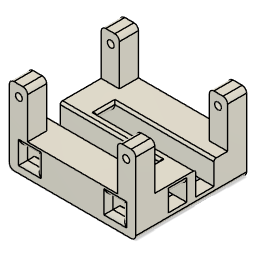
servoFrameMaking (Autodesk Fusion 360 design; units mm, degrees)
Autodesk Fusion 360 part; units mm, degrees
sketch "Sketch1" plane through (0, 0, 0) normal (1, 0, 0) x (0, 0, -1)
  line L0 (0, 0) -> (0, 7)
  line L1 (0, 7) -> (-1, 7)
  line L2 (-1, 7) -> (-1, 1.8)
  line L3 (-1, 1.8) -> (-5, 1.8)
  line L4 (-5, 1.8) -> (-5, 7)
  line L5 (-5, 7) -> (-12.2, 7)
  line L6 (-12.2, 7) -> (-12.2, 0)
  line L7 (-12.2, 0) -> (0, 0)
  dimension "d1" = 7
  dimension "d2" = 1
  dimension "d3" = 5.2
  dimension "d4" = 4
  dimension "d5" = 5.2
  dimension "d6" = 7.2
  dimension "d7" = 7
  constraint coincident L0.start L7.end
  constraint vertical L0
  constraint perpendicular L0 L1
  constraint perpendicular L1 L2
  constraint perpendicular L2 L3
  constraint perpendicular L3 L4
  constraint perpendicular L4 L5
  constraint perpendicular L5 L6
  measures "d1" distance of L0.start L0.end
  measures "d2" distance of L0.end L1.end
  measures "d3" distance of L1.end L2.end
  measures "d4" distance of L2.end L3.end
  measures "d5" distance of L3.end L4.end
  measures "d6" distance of L4.end L5.end
  measures "d7" distance of L5.end L6.end
extrude "Extrude1" add sketch "Sketch1" along normal blind 13.9 and the other way blind 13.9 makes body 1
sketch "Sketch2" plane through (0, 7, 0) normal (0, 1, 0) x (-1, 0, 0)
  line L0 (13.9, 12.2) -> (-13.9, 12.2)
  line L1 (-13.9, 12.2) -> (-13.9, 5)
  line L2 (-13.9, 5) -> (13.9, 5)
  line L3 (13.9, 5) -> (13.9, 12.2)
  line L4 (13.9, 12.2) -> (9.9, 12.2)
  line L5 (9.9, 12.2) -> (9.9, 8)
  line L6 (9.9, 8) -> (13.9, 8)
  line L7 (13.9, 8) -> (13.9, 12.2)
  dimension "d12" = 4
  dimension "d13" = 4.2
  constraint horizontal L4
  constraint vertical L5
  constraint horizontal L6
  constraint vertical L7
  constraint coincident L0.start L3.end
  measures "d12" distance of L0.start L4.end
  measures "d13" distance of L0.start L6.end
extrude "Extrude2" add sketch "Sketch2" along normal blind 10 separate body contours L0 L3 L4 L5 L6 L7 makes body 2
sketch "Sketch3" plane through (0, 0, 12.2) normal (0, 0, 1) x (1, 0, 0)
  line L0 (-13.9, 7) -> (-9.9, 7)
  line L1 (-9.9, 7) -> (-9.9, 17)
  line L2 (-9.9, 17) -> (-13.9, 17)
  line L3 (-13.9, 17) -> (-13.9, 7)
  line L4 (-13.9, 7) -> (-11.8, 7) construction
  line L5 (-11.8, 7) -> (-11.8, 14.6) construction
  line L6 (-11.8, 14.6) -> (-13.9, 14.6) construction
  line L7 (-13.9, 14.6) -> (-13.9, 7) construction
  circle A0 centre (-11.8, 14.6) radius 0.75
  dimension "d16" = 2.1
  dimension "d17" = 7.6
  dimension "d18" = 1.5
  constraint horizontal L4
  constraint vertical L5
  constraint horizontal L6
  constraint vertical L7
  constraint coincident L0.start L3.end
  constraint coincident L5.end L6.start
  measures "d16" distance of L0.start L4.end
  measures "d17" distance of L0.start L6.end
  measures "d18" diameter of A0
extrude "Extrude3" cut sketch "Sketch3" against normal blind 10 contours A0 bodies 2
fillet "Fillet1" radius 1 1 edges at (-13.9, 17, 10.1) on bodies 2
fillet "Fillet2" radius 1 1 edges at (-9.9, 17, 10.1) on bodies 2
mirror "Mirror1" about plane through (0, 0, 0) normal (1, 0, 0) of bodies 2 makes body 3
sketch "Sketch4" plane through (0, 0, 5) normal (0, 0, -1) x (-1, 0, 0)
  line L0 (13.9, 7) -> (-13.9, 7)
  line L1 (-13.9, 7) -> (-13.9, 1.8)
  line L2 (-13.9, 1.8) -> (13.9, 1.8)
  line L3 (13.9, 1.8) -> (13.9, 7)
  line L4 (-13.9, 7) -> (-7.9, 7)
  line L5 (-7.9, 7) -> (-7.9, 6.5)
  line L6 (-9.4, 5) -> (-12.4, 5)
  line L7 (-13.9, 6.5) -> (-13.9, 7)
  arc A0 (-9.4, 5) -> (-7.9, 6.5) centre (-9.4, 6.5) ccw
  arc A1 (-13.9, 6.5) -> (-12.4, 5) centre (-12.4, 6.5) ccw
  point P0 (-13.9, 5)
  dimension "d27" = 6
  dimension "d28" = 2
  dimension "d29" = 1.5
  dimension "d30" = 1.5
  constraint horizontal L4
  constraint vertical L5
  constraint horizontal L6
  constraint vertical L7
  constraint coincident L0.end L1.start
  constraint tangent L5 A0
  constraint tangent L6 A0
  constraint coincident P0 L6
  constraint coincident P0 L7
  constraint tangent L6 A1
  constraint tangent L7 A1
  measures "d27" distance of L0.end L4.end
  measures "d28" distance of L0.end P0
  measures "d29" radius of A0
  measures "d30" radius of A1
extrude "Extrude4" add sketch "Sketch4" along normal blind 4 contours L0 L1 L4 L5 L6 L7 A0 A1 bodies 1
sketch "Sketch5" plane through (13.9, 0, 0) normal (1, 0, 0) x (0, 0, -1)
  line L0 (0, 7) -> (-12.2, 7)
  line L1 (-12.2, 7) -> (-12.2, 0)
  line L2 (-12.2, 0) -> (0, 0)
  line L3 (0, 0) -> (0, 7)
  line L4 (-5, 6.5) -> (-1, 6.5)
  line L5 (-1, 6.5) -> (-1, 1.8)
  line L6 (-1, 1.8) -> (-5, 1.8)
  line L7 (-5, 1.8) -> (-5, 6.5)
  line L8 (-1, 1.8) -> (0, 1.8)
  line L9 (-5, 1.8) -> (-6, 1.8)
  line L10 (-12.2, 0) -> (-12.2, 2.5) construction
  line L11 (-12.2, 2.5) -> (-9.7, 2.5)
  line L12 (-12.2, 2.5) -> (-12.2, 5.5)
  line L13 (-12.2, 5.5) -> (-9.7, 5.5)
  line L14 (-9.7, 5.5) -> (-6, 1.8)
  line L15 (-12.2, 0) -> (-7, 0) construction
  line L16 (-9.7, 2.5) -> (-7, 0)
  dimension "d33" = 1
  dimension "d34" = 2.5
  dimension "d35" = 2.5
  dimension "d36" = 3
  dimension "d37" = 2.5
  dimension "d38" = 5.2
  constraint coincident L5.end L6.start
  constraint coincident L3 L8.end
  constraint perpendicular L3 L8
  constraint coincident L6.end L7.start
  constraint perpendicular L7 L9
  constraint coincident L1.end L2.start
  constraint perpendicular L2 L10
  constraint perpendicular L1 L11
  constraint perpendicular L11 L12
  constraint perpendicular L1 L13
  constraint perpendicular L5 L15
  measures "d33" distance of L6.end L9.end
  measures "d34" distance of L1.end L10.end
  measures "d35" distance of L10.end L11.end
  measures "d36" distance of L10.end L12.end
  measures "d37" distance of L12.end L13.end
  measures "d38" distance of L1.end L15.end
extrude "Extrude5" cut sketch "Sketch5" against normal blind 3 from surface at -3 contours L1 L2 L3 L6 L8 L9 L11 L12 L13 L14 L16 bodies 1
sketch "Sketch6" plane through (-13.9, 0, 0) normal (-1, 0, 0) x (0, 0, 1)
  line L0 (0, 0) -> (12.2, 0)
  line L1 (12.2, 0) -> (12.2, 7)
  line L2 (12.2, 7) -> (5, 7)
  line L3 (5, 7) -> (5, 1.8)
  line L4 (5, 1.8) -> (1, 1.8)
  line L5 (1, 1.8) -> (1, 7)
  line L6 (1, 7) -> (0, 7)
  line L7 (0, 7) -> (0, 0)
  line L8 (1, 1.8) -> (0, 1.8)
  line L9 (5, 1.8) -> (6, 1.8)
  line L10 (12.2, 0) -> (12.2, 2.5) construction
  line L11 (12.2, 2.5) -> (12.2, 5.5)
  line L12 (12.2, 5.5) -> (9.7, 5.5)
  line L13 (12.2, 2.5) -> (9.7, 2.5)
  line L14 (9.7, 5.5) -> (6, 1.8)
  line L15 (12.2, 0) -> (7, 0) construction
  line L16 (9.7, 2.5) -> (7, 0)
  dimension "d43" = 1
  dimension "d44" = 2.5
  dimension "d45" = 3
  dimension "d46" = 2.5
  dimension "d47" = 2.5
  dimension "d48" = 5.2
  constraint coincident L4.end L5.start
  constraint coincident L7 L8.end
  constraint perpendicular L7 L8
  constraint coincident L3.end L4.start
  constraint perpendicular L3 L9
  constraint coincident L0.end L1.start
  constraint coincident L1 L10.end
  constraint parallel L1 L11
  constraint perpendicular L1 L12
  constraint perpendicular L1 L13
  constraint perpendicular L10 L15
  measures "d43" distance of L3.end L9.end
  measures "d44" distance of L0.end L10.end
  measures "d45" distance of L10.end L11.end
  measures "d46" distance of L11.end L12.end
  measures "d47" distance of L10.end L13.end
  measures "d48" distance of L0.end L15.end
extrude "Extrude6" cut sketch "Sketch6" against normal blind 3 from surface at -3 contours L0 L1 L4 L7 L8 L9 L11 L12 L13 L14 L16 bodies 1
fillet "Fillet3" radius 0.5 3 edges at (-3, 7, 5) (7.9, 7, 3) (-3, 7, 1) on bodies 1
fillet "Fillet4" radius 1 1 edges at (13.9, 0, 6.1) on bodies 1
fillet "Fillet5" radius 1 1 edges at (-13.9, 0, 6.1) on bodies 1
fillet "Fillet6" radius 1 8 edges at (-9.4, 5.5, 12.2) (-7.9, 4, 12.2) (-9.4, 2.5, 12.2) (-10.9, 4, 12.2) (9.4, 5.5, 12.2) (10.9, 4, 12.2) (9.4, 2.5, 12.2) (7.9, 4, 12.2) on bodies 1
combine "Combine1" operation add target body 1 tool bodies 2 3
pattern_circular "C-Pattern1" count 1 over 360 about axis through (0, 1.75, 0) along (0, 1, 0) of bodies 1 merged
pattern_circular "C-Pattern2" count 2 over 360 about axis through (0, 1.75, 0) along (0, 1, 0) of bodies 1 makes body 4
combine "Combine2" operation add target body 1 tool bodies 4
